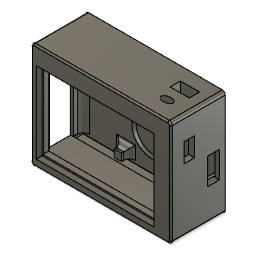
Rasp35inch_housing (Autodesk Fusion 360 design; units mm, degrees)
Autodesk Fusion 360 part; units mm, degrees
sketch "Skizze1" plane through (0, 0, 0) normal (0, 0, 1) x (1, 0, 0)
  line L0 (47.5, 36) -> (-47.5, 36)
  line L1 (-47.5, 36) -> (-47.5, -36)
  line L2 (-47.5, -36) -> (47.5, -36)
  line L3 (47.5, -36) -> (47.5, 36)
  line L4 (47.5, 36) -> (-47.5, -36) construction
  line L5 (-47.5, 36) -> (47.5, -36) construction
  dimension "d1" = 95
  dimension "d2" = 72
  constraint horizontal L0
  constraint perpendicular L0 L1
  constraint parallel L0 L2
  constraint parallel L1 L3
  constraint coincident L4 origin
  constraint coincident L5 origin
  measures "d1" distance of L0.start L0.end
  measures "d2" distance of L0.start L2.end
extrude "Extrusion1" add sketch "Skizze1" along normal blind 40 makes body 1
sketch "Skizze2" plane through (0, 0, 0) normal (0, 0, -1) x (-1, 0, 0)
  line L0 (-47.5, 36) -> (-47.5, -36)
  line L1 (-47.5, -36) -> (47.5, -36)
  line L2 (47.5, -36) -> (47.5, 36)
  line L3 (47.5, 36) -> (-47.5, 36)
  line L4 (42, -29) -> (-34, -29)
  line L5 (-34, -29) -> (-34, 22)
  line L6 (-34, 22) -> (42, 22)
  line L7 (42, 22) -> (42, -29)
  line L8 (42, -29) -> (-34, 22) construction
  line L9 (-34, -29) -> (42, 22) construction
  point P0 (4, -3.5)
  dimension "d5" = 76
  dimension "d6" = 51
  dimension "d8" = 7
  dimension "d81" = 5.5
  constraint horizontal L4
  constraint perpendicular L4 L5
  constraint parallel L4 L6
  constraint parallel L5 L7
  constraint coincident L8 P0
  constraint coincident L9 P0
  measures "d5" distance of L5.end L6.end
  measures "d6" distance of L4.end L5.end
  measures "d8" distance of L1 L4
  measures "d81" distance of L2 L7
extrude "Extrusion2" cut sketch "Skizze2" against normal blind 70 contours L4 L5 L6 L7 bodies 1
sketch "Skizze3" plane through (0, 0, 0) normal (0, 0, -1) x (-1, 0, 0)
  line L0 (-34, -29) -> (-34, 22)
  line L1 (-34, 22) -> (42, 22)
  line L2 (42, 22) -> (42, -29)
  line L3 (42, -29) -> (-34, -29)
  line L4 (-47.5, 36) -> (-47.5, -36)
  line L5 (-47.5, -36) -> (47.5, -36)
  line L6 (47.5, -36) -> (47.5, 36)
  line L7 (47.5, 36) -> (-47.5, 36)
  line L8 (-41.5, 25) -> (44.5, 25)
  line L9 (44.5, 25) -> (44.5, -31)
  line L10 (44.5, -31) -> (-41.5, -31)
  line L11 (-41.5, -31) -> (-41.5, 25)
  line L12 (-41.5, 25) -> (44.5, -31) construction
  line L13 (44.5, 25) -> (-41.5, -31) construction
  point P0 (1.5, -3)
  dimension "d11" = 86
  dimension "d12" = 3
  dimension "d13" = 56
  dimension "d14" = 5
  constraint horizontal L8
  constraint perpendicular L8 L9
  constraint parallel L8 L10
  constraint parallel L9 L11
  constraint coincident L12 P0
  constraint coincident L13 P0
  measures "d11" distance of L8.start L8.end
  measures "d12" distance of L6 L9
  measures "d13" distance of L8.end L9.end
  measures "d14" distance of L5 L10
extrude "Extrusion3" cut sketch "Skizze3" against normal blind 37 contours L8 L9 L10 L11 bodies 1
sketch "Skizze4" plane through (0, 0, 0) normal (0, 0, -1) x (-1, 0, 0)
  line L0 (44.5, 25) -> (44.5, -31)
  line L1 (44.5, -31) -> (-41.5, -31)
  line L2 (-41.5, -31) -> (-41.5, 25)
  line L3 (-41.5, 25) -> (44.5, 25)
  line L4 (-47.5, 36) -> (-47.5, -36)
  line L5 (-47.5, -36) -> (47.5, -36)
  line L6 (47.5, -36) -> (47.5, 36)
  line L7 (47.5, 36) -> (-47.5, 36)
  line L8 (-43.5, 25) -> (46, 25)
  line L9 (46, 25) -> (46, -32)
  line L10 (46, -32) -> (-43.5, -32)
  line L11 (-43.5, -32) -> (-43.5, 25)
  dimension "d18" = 2
  dimension "d20" = 1.5
  dimension "d21" = 1
  constraint horizontal L8
  constraint vertical L9
  constraint horizontal L10
  constraint vertical L11
  constraint collinear L3 L8
  measures "d18" distance of L2 L11
  measures "d20" distance of L0 L9
  measures "d21" distance of L1 L10
extrude "Extrusion4" cut sketch "Skizze4" along normal blind 45 from surface at -31 contours L0 L1 L2 L8 L9 L10 L11 bodies 1
sketch "Skizze5" plane through (0, 0, 0) normal (0, 0, -1) x (-1, 0, 0)
  line L0 (46, -32) -> (-43.5, -32)
  line L1 (-43.5, -32) -> (-43.5, 25)
  line L2 (-43.5, 25) -> (46, 25)
  line L3 (46, 25) -> (46, -32)
  line L4 (-47.5, 36) -> (-47.5, -36)
  line L5 (-47.5, -36) -> (47.5, -36)
  line L6 (47.5, -36) -> (47.5, 36)
  line L7 (47.5, 36) -> (-47.5, 36)
  line L8 (-19, 34.5) -> (-2, 34.5)
  line L9 (-2, 34.5) -> (-2, 25)
  line L10 (-2, 25) -> (-19, 25)
  line L11 (-19, 25) -> (-19, 34.5)
  line L12 (46, 25) -> (44.5, 25)
  line L13 (7, 25) -> (14, 25)
  line L14 (14, 25) -> (14, 28)
  line L15 (14, 28) -> (7, 28)
  line L16 (7, 28) -> (7, 25)
  line L17 (-36.5, 25) -> (-28.5, 25)
  line L18 (-28.5, 25) -> (-28.5, 28)
  line L19 (-28.5, 28) -> (-36.5, 28)
  line L20 (-36.5, 28) -> (-36.5, 25)
  line L21 (-43.5, 25) -> (-41.5, 25)
  dimension "d26" = 9.5
  dimension "d27" = 17
  dimension "d31" = 9
  dimension "d32" = 7
  dimension "d33" = 3
  dimension "d35" = 8
  dimension "d36" = 3
  dimension "d82" = 28.5
  dimension "d83" = 11
  constraint horizontal L8
  constraint vertical L9
  constraint horizontal L10
  constraint vertical L11
  constraint collinear L10 L12
  constraint horizontal L13
  constraint vertical L14
  constraint horizontal L15
  constraint vertical L16
  constraint coincident L12 L13.start
  constraint horizontal L17
  constraint vertical L18
  constraint horizontal L19
  constraint vertical L20
  constraint coincident L12 L17.start
  measures "d26" distance of L8.end L9.end
  measures "d27" distance of L8.start L8.end
  measures "d31" distance of L9 L16
  measures "d32" distance of L14.end L15.end
  measures "d33" distance of L13.end L14.end
  measures "d35" distance of L18.end L19.end
  measures "d36" distance of L17.end L18.end
  measures "d82" distance of L4 L11
  measures "d83" distance of L4 L20
extrude "Extrusion5" cut sketch "Skizze5" along normal blind 36 from surface at -31 contours L2 L13 L14 L15 L16 | L2 L17 L18 L19 L20 | L2 L8 L9 L10 L11 bodies 1
sketch "Skizze6" plane through (0, 28, 0) normal (0, -1, 0) x (1, 0, 0)
  line L0 (28.5, 0) -> (36.5, 0)
  line L1 (36.5, 0) -> (36.5, 31)
  line L2 (36.5, 31) -> (28.5, 31)
  line L3 (28.5, 31) -> (28.5, 0)
  ellipse E0 centre (32.5, 27.5) end of major axis (36.5, 27.5) minor radius 2.5
  line L4 (28.5, 27.5) -> (36.5, 27.5)
  line L5 (32.5, 25) -> (32.5, 30)
  line L6 (39, 19) -> (26, 19)
  line L7 (26, 19) -> (26, 12)
  line L8 (26, 12) -> (39, 12)
  line L9 (39, 12) -> (39, 19)
  line L10 (39, 19) -> (26, 12) construction
  line L11 (26, 19) -> (39, 12) construction
  line L12 (36.5, 31) -> (28.5, 31)
  point P0 (32.5, 15.5)
  dimension "d37" = 5
  dimension "d46" = 13
  dimension "d47" = 7
  dimension "d48" = 12
  dimension "d86" = 3.5
  constraint parallel L2 L4
  constraint coincident E0 L4.start
  constraint coincident E0 L4.end
  constraint coincident E0 L5.start
  constraint coincident E0 L5.end
  constraint coincident L1 L4.end
  constraint coincident L3 L4.start
  constraint horizontal L6
  constraint perpendicular L6 L7
  constraint parallel L6 L8
  constraint parallel L7 L9
  constraint coincident L10 P0
  constraint coincident L11 P0
  constraint vertical E0.centre P0
  measures "d46" distance of L6.start L6.end
  measures "d47" distance of L6.start L8.end
  measures "d48" distance of E0.centre P0
  measures "d86" distance of L4 L12
extrude "Extrusion6" cut sketch "Skizze6" along normal blind -11 and the other way blind -8 contours L3 L6 L7 L8 | L1 L3 L6 L8 | L1 L6 L8 L9 | E0 L4 L5 | E0 L4 L5 | E0 L4 L5 | E0 L4 L5 bodies 1
sketch "Skizze7" plane through (43.5, 0, 0) normal (-1, 0, 0) x (0, 0, 1)
  line L0 (0, 25) -> (0, -32)
  line L1 (0, -32) -> (31, -32)
  line L2 (31, -32) -> (31, 25)
  line L3 (31, 25) -> (0, 25)
  line L4 (31, 20.5) -> (24, 20.5)
  line L5 (24, 20.5) -> (24, 7.5)
  line L6 (24, 7.5) -> (31, 7.5)
  line L7 (31, 7.5) -> (31, 20.5)
  dimension "d41" = 4.5
  dimension "d42" = 13
  dimension "d43" = 7
  constraint horizontal L4
  constraint vertical L5
  constraint horizontal L6
  constraint vertical L7
  constraint coincident L2 L4.start
  measures "d41" distance of L3 L4
  measures "d42" distance of L4.end L5.end
  measures "d43" distance of L5.end L6.end
extrude "Extrusion7" cut sketch "Skizze7" against normal blind 8 contours L2 L4 L5 L6 L7 bodies 1
sketch "Skizze8" plane through (0, 0, 0) normal (0, 0, -1) x (-1, 0, 0)
  line L0 (-2, 34.5) -> (-2, 25)
  line L1 (-2, 25) -> (7, 25)
  line L2 (7, 25) -> (7, 28)
  line L3 (7, 28) -> (14, 28)
  line L4 (14, 28) -> (14, 25)
  line L5 (46, 25) -> (46, -32)
  line L6 (46, -32) -> (-43.5, -32)
  line L7 (-43.5, -32) -> (-43.5, 25)
  line L8 (-36.5, 25) -> (-36.5, 28)
  line L9 (-36.5, 28) -> (-28.5, 28)
  line L10 (-28.5, 28) -> (-28.5, 25)
  line L11 (-19, 25) -> (-19, 34.5)
  line L12 (-19, 34.5) -> (-2, 34.5)
  line L13 (-47.5, 36) -> (-47.5, -36)
  line L14 (-47.5, -36) -> (47.5, -36)
  line L15 (47.5, -36) -> (47.5, 36)
  line L16 (47.5, 36) -> (-47.5, 36)
  line L17 (-43.5, 26) -> (46, 26)
  line L18 (46, 26) -> (46, -34)
  line L19 (46, -34) -> (-43.5, -34)
  line L20 (-43.5, -34) -> (-43.5, 26)
  line L21 (14, 25) -> (46, 25)
  line L22 (-43.5, 25) -> (-36.5, 25)
  line L23 (-28.5, 25) -> (-19, 25)
  dimension "d51" = 2
  constraint horizontal L17
  constraint vertical L18
  constraint horizontal L19
  constraint vertical L20
  constraint collinear L7 L20
  constraint collinear L5 L18
  measures "d51" distance of L6 L19
extrude "Extrusion8" cut sketch "Skizze8" along normal blind 35 from surface at -13 contours L6 L18 L19 L20 bodies 1
sketch "Skizze9" plane through (-46, 0, 0) normal (1, 0, 0) x (0, 0, -1)
  line L0 (0, -34) -> (0, 25)
  line L1 (0, 25) -> (-31, 25)
  line L2 (-31, 25) -> (-31, -32)
  line L3 (-31, -32) -> (-13, -32)
  line L4 (-13, -32) -> (-13, -34)
  line L5 (-13, -34) -> (0, -34)
  line L6 (-31, 21) -> (0, 21)
  line L7 (0, 21) -> (0, -32)
  line L8 (0, -32) -> (-31, -32)
  line L9 (-31, -32) -> (-31, 21)
  line L10 (-29, 21) -> (-29, -32)
  point P0 (0, -36)
  dimension "d56" = 53
  dimension "d85" = 4
  dimension "d87" = 2
  constraint horizontal L6
  constraint vertical L7
  constraint horizontal L8
  constraint vertical L9
  constraint coincident L0 L7.end
  constraint coincident L2 L6.start
  constraint coincident L6 L10.start
  constraint coincident L8 L10.end
  constraint perpendicular L8 L10
  measures "d56" distance of L6.end L7.end
  measures "d85" distance of L7.end P0
  measures "d87" distance of L9 L10
extrude "Extrusion9" cut sketch "Skizze9" against normal blind 3 contours L0 L3 L6 L7 L8 L10 bodies 1
sketch "Skizze10" plane through (0, 0, 0) normal (0, 0, -1) x (-1, 0, 0)
  line L0 (46, 21) -> (47.5, 21)
  line L1 (47.5, 21) -> (47.5, 36)
  line L2 (47.5, 36) -> (-47.5, 36)
  line L3 (-47.5, 36) -> (-47.5, -36)
  line L4 (-47.5, -36) -> (47.5, -36)
  line L5 (47.5, -32) -> (46, -32)
  line L6 (46, -32) -> (46, -34)
  line L7 (46, -34) -> (-43.5, -34)
  line L8 (-43.5, -34) -> (-43.5, 25)
  line L9 (-36.5, 25) -> (-36.5, 28)
  line L10 (-36.5, 28) -> (-28.5, 28)
  line L11 (-28.5, 28) -> (-28.5, 25)
  line L12 (-19, 25) -> (-19, 34.5)
  line L13 (-19, 34.5) -> (-2, 34.5)
  line L14 (-2, 34.5) -> (-2, 25)
  line L15 (7, 25) -> (7, 28)
  line L16 (7, 28) -> (14, 28)
  line L17 (14, 28) -> (14, 25)
  line L18 (-46, 34.5) -> (46, 34.5)
  line L19 (46, 34.5) -> (46, -34.5)
  line L20 (-46, -34.5) -> (-46, 34.5)
  line L21 (-46, -34.5) -> (46, -34.5)
  line L22 (-43.5, 25) -> (-36.5, 25)
  line L23 (-2, 25) -> (7, 25)
  line L24 (14, 25) -> (46, 25)
  line L25 (-28.5, 25) -> (-19, 25)
  line L26 (46, 25) -> (46, 21)
  line L27 (47.5, -36) -> (47.5, -32)
  dimension "d59" = 1.5
  dimension "d60" = 1.5
  dimension "d61" = 1.5
  constraint horizontal L18
  constraint vertical L19
  constraint vertical L20
  constraint perpendicular L19 L21
  measures "d59" distance of L2 L18
  measures "d60" distance of L3 L20
  measures "d61" distance of L4 L21
extrude "Extrusion10" cut sketch "Skizze10" against normal blind 6 contours L14 L15 L16 L17 L18 L19 L23 L24 | L7 L8 L9 L10 L11 L12 L18 L19 L20 L21 L22 L25 bodies 1
extrude "Extrusion11" cut 1 faces at (15.3333, -35.5, 0) along direction (0, 0, 1) blind 3 on bodies 1 bodies 1
fillet "Abrundung1" radius 2 4 edges at (-47.5, -36, 21.5) (-47.5, 36, 21.5) (47.5, 36, 21.5) (47.5, -36, 21.5) on bodies 1
chamfer "Fase1" distance 2 angle 45 4 edges at (-4, 22, 40) (-42, -3.5, 40) (34, -3.5, 40) (-4, -29, 40) on bodies 1
fillet "Abrundung2" radius 1 8 edges at (46.9142, -35.4142, 40) (47.5, 0, 40) (46.9142, 35.4142, 40) (0, 36, 40) (-46.9142, 35.4142, 40) (-47.5, 0, 40) (-46.9142, -35.4142, 40) (0, -36, 40) on bodies 1
sketch "Skizze11" plane through (43.5, 0, 0) normal (-1, 0, 0) x (0, 0, 1)
  line L0 (6, 25) -> (6, -34)
  line L1 (6, -34) -> (13, -34)
  line L2 (13, -34) -> (13, -32)
  line L3 (13, -32) -> (31, -32)
  line L4 (31, -32) -> (31, 7.5)
  line L5 (31, 7.5) -> (24, 7.5)
  line L6 (24, 7.5) -> (24, 20.5)
  line L7 (24, 20.5) -> (31, 20.5)
  line L8 (31, 25) -> (6, 25)
  line L9 (9, 2) -> (13, 2)
  line L10 (13, 2) -> (13, -12)
  line L11 (13, -12) -> (9, -12)
  line L12 (9, -12) -> (9, 2)
  line L13 (31, 20.5) -> (31, 25)
  dimension "d72" = 14
  dimension "d73" = 22
  dimension "d74" = 4
  dimension "d84" = 3
  constraint horizontal L9
  constraint vertical L10
  constraint horizontal L11
  constraint vertical L12
  measures "d72" distance of L9.start L11.end
  measures "d73" distance of L1 L11
  measures "d74" distance of L9.start L9.end
  measures "d84" distance of L0 L12
extrude "Extrusion12" cut sketch "Skizze11" against normal blind 8 contours L9 L10 L11 L12 bodies 1
chamfer "Fase2" distance 2 angle 45 4 edges at (47.5, -5, 13) (47.5, -5, 9) (47.5, -12, 11) (47.5, 2, 11) on bodies 1
sketch "Skizze12" plane through (0, 0, 6) normal (0, 0, -1) x (-1, 0, 0)
  line L0 (-46, 34.5) -> (-46, -34.5)
  line L1 (-46, -34.5) -> (46, -34.5)
  line L2 (46, -34.5) -> (46, -34)
  line L3 (46, -34) -> (-43.5, -34)
  line L4 (-43.5, -34) -> (-43.5, 25)
  line L5 (-43.5, 25) -> (-36.5, 25)
  line L6 (-36.5, 25) -> (-36.5, 28)
  line L7 (-36.5, 28) -> (-28.5, 28)
  line L8 (-28.5, 28) -> (-28.5, 25)
  line L9 (-28.5, 25) -> (-19, 25)
  line L10 (-19, 25) -> (-19, 34.5)
  line L11 (-19, 34.5) -> (-46, 34.5)
  line L12 (-43.5, 2) -> (-46, 2)
  line L13 (-46, 2) -> (-46, -12)
  line L14 (-46, -12) -> (-43.5, -12)
  line L15 (-43.5, -12) -> (-43.5, 2)
  line L16 (-43.5, 2) -> (-43.5, -12)
  dimension "d78" = 2.5
  constraint horizontal L12
  constraint vertical L13
  constraint horizontal L14
  constraint vertical L15
  constraint coincident L4 L12.start
  constraint coincident L12.start L15.end
  constraint coincident L14.end L15.start
  measures "d78" distance of L12.start L12.end
extrude "Extrusion13" cut sketch "Skizze12" against normal blind 5 contours L0 L4 L12 L13 L14 L15 L16 bodies 1
extrude "Extrusion14" cut 1 faces at (13.3333, 28.1667, 31) along direction (0, 0, 1) blind 2 on bodies 1 bodies 1
sketch "Skizze1 (2)" plane through (0, 0, 6) normal (0, 0, -1) x (-1, 0, 0) in component "Deckel"
  line L0 (-46, 2) -> (-43.5, 2) construction
  line L1 (-43.5, 2) -> (-43.5, 25) construction
  line L2 (-43.5, 25) -> (-36.5, 25) construction
  line L3 (-36.5, 25) -> (-36.5, 28) construction
  line L4 (-36.5, 28) -> (-28.5, 28) construction
  line L5 (-28.5, 28) -> (-28.5, 25) construction
  line L6 (-28.5, 25) -> (-19, 25) construction
  line L7 (-19, 25) -> (-19, 34.5) construction
  line L8 (-19, 34.5) -> (-46, 34.5) construction
  line L9 (-46, 34.5) -> (-46, 2) construction
  line L10 (46, 34.5) -> (-46, 34.5) construction
  line L11 (-46, 34.5) -> (-46, -34.5) construction
  line L12 (46, 21) -> (46, 34.5) construction
  line L13 (46, -34.5) -> (46, -32) construction
  line L14 (-46, -34.5) -> (46, -34.5) construction
  line L15 (-45.75, 34.25) -> (45.75, 34.25)
  line L16 (45.75, 34.25) -> (45.75, -34.25)
  line L17 (45.75, -34.25) -> (-45.75, -34.25)
  line L18 (-45.75, -34.25) -> (-45.75, 34.25)
  dimension "d90" = 0.25
  dimension "d91" = 0.25
  dimension "d92" = 0.25
  dimension "d93" = 0.25
  constraint horizontal L15
  constraint vertical L16
  constraint horizontal L17
  constraint vertical L18
  measures "d90" distance of L10 L15
  measures "d91" distance of L9 L18
  measures "d92" distance of L14 L17
  measures "d93" distance of L12 L16
extrude "Extrusion1'" add sketch "Skizze1 (2)" along normal blind 2.5 separate body makes body 2 in component "Deckel"
sketch "Skizze3 (2)" plane through (0, 0, 6) normal (0, 0, 1) x (1, 0, 0) in component "Deckel"
  line L0 (-45.75, -34.25) -> (45.75, -34.25)
  line L1 (45.75, -34.25) -> (45.75, 34.25)
  line L2 (45.75, 34.25) -> (-45.75, 34.25)
  line L3 (-45.75, 34.25) -> (-45.75, -34.25)
  line L4 (36.5, 25) -> (43.5, 25)
  line L5 (43.5, 25) -> (43.5, 2)
  line L6 (43.5, -12) -> (43.5, -34)
  line L7 (43.5, -32) -> (-46, -32)
  line L8 (43.5, -34) -> (-46, -34)
  line L9 (43.5, -32) -> (38.5, -32)
  line L10 (38.5, -32) -> (38.5, -27)
  line L11 (38.5, -27) -> (43.5, -27)
  line L12 (43.5, -27) -> (43.5, -32)
  line L13 (43.5, 25) -> (38.5, 25)
  line L14 (38.5, 25) -> (38.5, 20)
  line L15 (38.5, 20) -> (43.5, 20)
  line L16 (43.5, 20) -> (43.5, 25)
  line L17 (-19.5, 25) -> (-14.5, 25)
  line L18 (-14.5, 25) -> (-14.5, 20)
  line L19 (-14.5, 20) -> (-19.5, 20)
  line L20 (-19.5, 20) -> (-19.5, 25)
  line L21 (-19.5, -32) -> (-14.5, -32)
  line L22 (-14.5, -32) -> (-14.5, -27)
  line L23 (-14.5, -27) -> (-19.5, -27)
  line L24 (-19.5, -27) -> (-19.5, -32)
  dimension "d96" = 5
  dimension "d97" = 5
  dimension "d98" = 58
  constraint horizontal L9
  constraint vertical L10
  constraint horizontal L11
  constraint vertical L12
  constraint coincident L7.start L9.start
  constraint equal L10 L11
  constraint horizontal L13
  constraint vertical L14
  constraint horizontal L15
  constraint vertical L16
  constraint coincident L4.end L5.start
  constraint collinear L10 L14
  constraint horizontal L17
  constraint vertical L18
  constraint horizontal L19
  constraint vertical L20
  constraint horizontal L21
  constraint vertical L22
  constraint horizontal L23
  constraint vertical L24
  constraint coincident L7 L21.start
  constraint collinear L11 L23
  constraint equal L11 L23
  constraint equal L19 L23
  constraint collinear L18 L22
  constraint collinear L13 L17
  constraint collinear L15 L19
  measures "d96" distance of L9.end L10.end
  measures "d97" distance of L4.end L15.end
  measures "d98" distance of L14 L20
extrude "Extrusion2'" add sketch "Skizze3 (2)" along normal blind 5.5 contours L7 L21 L22 L23 L24 | L6 L7 L9 L10 L11 L12 | L4 L5 L13 L14 L15 L16 | L17 L18 L19 L20 bodies 2 in component "Deckel"
fillet "Abrundung1'" radius 4 10 edges at (-17, 20, 6) (-14.5, 22.5, 6) (-19.5, 22.5, 6) (41, 20, 6) (38.5, 22.5, 6) (-19.5, -29.5, 6) (-14.5, -29.5, 6) (-17, -27, 6) (38.5, -29.5, 6) (41, -27, 6) on bodies 2 in component "Deckel"
sketch "Skizze4 (2)" plane through (-45.75, 0, 0) normal (-1, 0, 0) x (0, 0, 1) in component "Deckel"
  line L0 (6, -34.25) -> (6, 34.25)
  line L1 (6, 34.25) -> (3.5, 34.25)
  line L2 (3.5, 34.25) -> (3.5, -34.25)
  line L3 (3.5, -34.25) -> (6, -34.25)
  line L4 (3.5, 34.25) -> (6, 34.25)
  line L5 (6, 34.25) -> (6, -32.25)
  line L6 (6, -32.25) -> (3.5, -32.25)
  line L7 (3.5, -32.25) -> (3.5, 34.25)
  dimension "d103" = 2
  constraint horizontal L4
  constraint vertical L5
  constraint horizontal L6
  constraint vertical L7
  constraint coincident L0 L5.end
  constraint coincident L1.end L2.start
  measures "d103" distance of L3 L6
extrude "Extrusion3'" add sketch "Skizze4 (2)" along normal blind 2 contours L0 L1 L2 L4 L5 L6 L7 bodies 2 in component "Deckel"
sketch "Skizze5 (2)" plane through (0, 0, 6) normal (0, 0, 1) x (1, 0, 0) in component "Deckel"
  line L0 (-45.75, -34.25) -> (45.75, -34.25)
  line L1 (45.75, -34.25) -> (45.75, 34.25)
  line L2 (45.75, 34.25) -> (-45.75, 34.25)
  line L3 (-45.75, 34.25) -> (-45.75, -32.25)
  line L4 (-45.75, -32.25) -> (-45.75, -34.25)
  line L5 (-10.5, -32) -> (-23.5, -32)
  line L6 (-23.5, -32) -> (-23.5, -23)
  line L7 (-23.5, -23) -> (-10.5, -23)
  line L8 (-10.5, -23) -> (-10.5, -32)
  line L9 (43.5, 25) -> (43.5, 16)
  line L10 (43.5, 16) -> (34.5, 16)
  line L11 (34.5, 16) -> (34.5, 25)
  line L12 (34.5, 25) -> (43.5, 25)
  line L13 (43.5, -32) -> (34.5, -32)
  line L14 (34.5, -32) -> (34.5, -23)
  line L15 (34.5, -23) -> (43.5, -23)
  line L16 (43.5, -23) -> (43.5, -32)
  line L17 (-23.5, 25) -> (-10.5, 25)
  line L18 (-10.5, 25) -> (-10.5, 16)
  line L19 (-10.5, 16) -> (-23.5, 16)
  line L20 (-23.5, 16) -> (-23.5, 25)
  circle A0 centre (0.5, -12) radius 12
  line L21 (-19.5, 20) -> (-14.5, 20)
  line L22 (-14.5, 20) -> (-14.5, 25)
  line L23 (-14.5, -27) -> (-19.5, -27)
  dimension "d106" = 24
  dimension "d108" = 15
  dimension "d117" = 15
  measures "d106" diameter of A0
  measures "d108" distance of A0.centre L22
  measures "d117" distance of A0.centre L23
extrude "Extrusion4'" cut sketch "Skizze5 (2)" against normal blind 1.5 contours A0 bodies 2 in component "Deckel"
chamfer "Fase1'" distance 1.5 angle 45 1 edges at (-10.6879, -7.6606, 6) on bodies 2 in component "Deckel"
sketch "Skizze6 (2)" plane through (0, 0, 6) normal (0, 0, 1) x (1, 0, 0) in component "Deckel"
  line L0 (-45.75, -32.25) -> (-45.75, 34.25)
  line L1 (-45.75, 34.25) -> (-47.75, 34.25)
  line L2 (-47.75, 34.25) -> (-47.75, -32.25)
  line L3 (-47.75, -32.25) -> (-45.75, -32.25)
  line L4 (-47.75, -32.25) -> (-45.75, -32.25)
  line L5 (-45.75, -32.25) -> (-45.75, 20.75)
  line L6 (-45.75, 20.75) -> (-47.75, 20.75)
  line L7 (-47.75, 20.75) -> (-47.75, -32.25)
  dimension "d112" = 53
  constraint horizontal L4
  constraint vertical L5
  constraint horizontal L6
  constraint vertical L7
  constraint coincident L0 L5.end
  constraint coincident L2.end L3.start
  measures "d112" distance of L2.end L6.end
extrude "Extrusion5'" add sketch "Skizze6 (2)" along normal blind 7 contours L0 L2 L3 L4 L5 L6 L7 bodies 2 in component "Deckel"
fillet "Abrundung2'" radius 4 1 edges at (-45.75, -5.75, 6) on bodies 2 in component "Deckel"
component "Deckel" placed x (1, 0, 0) y (0, 1, 0) z (0, 0, 1) at (0, 0, 0)
equation "d16 = -40.00 mm + 3 mm"
equation "d60 = d59"
equation "d81 = 9.50 mm - 4 mm"
equation "d91 = d90"
equation "d92 = d90"
equation "d93 = d90"
equation "d97 = d96"
equation "d107 = 15 mm"
equation "d108 = d107"
equation "d113 = 5.5 mm + 1.5 mm"
